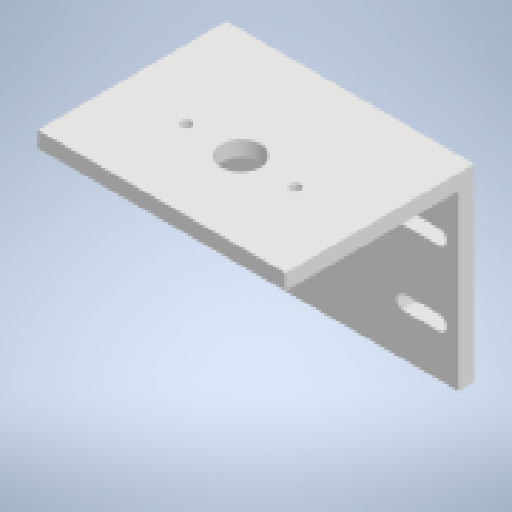
# Autodesk Inventor part: Suporte motor sensor
Saved by Autodesk Inventor 2023 (Build 270158000, 158)
## iProperties
Created: 2022-10-13
Part Number: Suporte motor sensor
Material: Generic
Document SubType Name: Modeling
Designer: klebe
Density: 1 g/cm^3
Appearance: Default
Author: klebe
Autodesk Inventor part; units mm, degrees
ref_plane "YZ Plane" through (0, 0, 0) normal (1, 0, 0) x (0, 1, 0)
ref_plane "XZ Plane" through (0, 0, 0) normal (0, 1, 0) x (-1, 0, 0)
ref_plane "XY Plane" through (0, 0, 0) normal (0, 0, 1) x (1, 0, 0)
sketch "Sketch1" plane through (0, 0, 0) normal (0, 0, 1) x (1, 0, 0)
  line L0 (-200, 100) -> (200, 100) projected
  line L1 (-200, -100) -> (-200, 100) projected
  line L2 (200, -100) -> (-200, -100) projected
  line L3 (121.9, 74) -> (121.9, 71)
  line L4 (171.9, 74) -> (121.9, 74)
  line L5 (171.9, 71) -> (171.9, 35.9)
  line L6 (121.9, 71) -> (171.9, 71)
  line L7 (121.9, 71) -> (121.9, 35.9)
  line L8 (171.9, 35.9) -> (121.9, 35.9)
  line L9 (171.9, 71) -> (171.9, 35.9)
  line L10 (171.9, 74) -> (171.9, 71)
  line L11 (121.9, 35.9) -> (171.9, 35.9)
  line L12 (171.9, 35.9) -> (171.9, 71)
  line L13 (171.9, 71) -> (121.9, 71)
  line L14 (121.9, 71) -> (121.9, 35.9)
  point P0 (0, 0)
  constraints: 24 end point, 2 parallel, 1 horizontal, 1 perpendicular
extrude "Extrusion1" add sketch "Sketch1" along normal blind 3.175
sketch "Sketch2" plane through (0, 0, 3.175) normal (0, 0, 1) x (1, 0, 0)
  line L0 (171.9, 74) -> (121.9, 74) projected
  line L1 (171.9, 35.9) -> (171.9, 74) projected
  line L2 (121.9, 74) -> (171.9, 74)
  line L3 (171.9, 74) -> (171.9, 71)
  line L4 (121.9, 71) -> (121.9, 74)
  line L5 (121.9, 71) -> (121.9, 70.825)
  line L6 (121.9, 74) -> (121.9, 35.9) projected
  line L7 (121.9, 70.825) -> (171.9, 70.825)
  line L8 (171.9, 71) -> (171.9, 70.825)
  line L9 (171.9, 71) -> (171.9, 70.825)
  point P0 (0, 0)
  dimension "d3" = 3
  dimension "d54" = 0.175
  constraints: 14 end point, 3 point on line, 2 collinear, 2 perpendicular, 1 horizontal, 1 parallel
  measures "d3" distance of L2.end L3.end
  measures "d54" distance of L4.start L5.end
extrude "Extrusion2" add sketch "Sketch2" along normal blind 34.925
sketch "Sketch3" plane through (121.9, 74, 0) normal (0, 1, 0) x (1, 0, 0)
  line L0 (50, 0) -> (0, 0) projected
  line L1 (0, 0) -> (0, -38.1) projected
  line L2 (50, -38.1) -> (0, -38.1) projected
  line L3 (50, 0) -> (50, -38.1) projected
  line L4 (50, -3.175) -> (50, -38.1) projected
  line L5 (0, -38.1) -> (0, -19.225)
  line L6 (50, -19.05) -> (60.9839, -19.05)
  line L7 (0, -38.1) -> (0, -22.1)
  line L8 (0, -22.1) -> (14, -22.1)
  line L9 (36, -22.1) -> (36, -22)
  point P0 (-121.9, 0)
  point P1 (14, -22)
  dimension "d55" = 16
  constraints: 10 end point, 4 point on line, 2 perpendicular, 1 vertical
  measures "d55" distance of L1.end L7.end
sketch "Sketch4" plane through (121.9, 74, 0) normal (0, 1, 0) x (1, 0, 0)
  line L0 (50, 0) -> (0, 0) projected
  line L1 (0, 0) -> (0, -38.1) projected
  line L2 (50, -38.1) -> (0, -38.1) projected
  line L3 (50, 0) -> (50, -38.1) projected
  line L4 (0, -38.1) -> (0, -22.1)
  line L5 (25, -22) -> (25, -22)
  point P0 (-121.9, 0)
  dimension "d56" = 16
  constraints: 4 end point, 1 point on line, 1 vertical
  measures "d56" distance of L1.end L4.end
hole "Hole2" at (146.9, 74, 22) direction (0, -1, 0) diameter 8 end through all
hole "Hole3" at (135.9, 74, 22.1) at (157.9, 74, 22.1) direction (0, -1, 0) diameter 2 end through all
sketch "Sketch5" plane through (0, 0, 3.175) normal (0, 0, 1) x (1, 0, 0)
  line L0 (121.9, 70.825) -> (121.9, 35.9) projected
  line L1 (121.9, 35.9) -> (171.9, 35.9) projected
  line L2 (171.9, 35.9) -> (171.9, 70.825) projected
  line L3 (171.9, 70.825) -> (121.9, 70.825) projected
  line L4 (121.9, 35.9) -> (171.9, 35.9) projected
  line L5 (171.9, 35.9) -> (167.9, 35.9)
  arc A0 (167.9, 44.31) -> (167.9, 47.49) centre (167.9, 45.9) ccw
  arc A1 (160.9, 47.49) -> (160.9, 44.31) centre (160.9, 45.9) ccw
  line L6 (167.9, 44.31) -> (160.9, 44.31)
  line L7 (160.9, 47.49) -> (167.9, 47.49)
  arc A2 (167.9, 59.31) -> (167.9, 62.49) centre (167.9, 60.9) ccw
  arc A3 (160.9, 62.49) -> (160.9, 59.31) centre (160.9, 60.9) ccw
  line L8 (167.9, 59.31) -> (160.9, 59.31)
  line L9 (160.9, 62.49) -> (167.9, 62.49)
  arc A4 (132.9, 44.31) -> (132.9, 47.49) centre (132.9, 45.9) ccw
  arc A5 (125.9, 47.49) -> (125.9, 44.31) centre (125.9, 45.9) ccw
  line L10 (132.9, 44.31) -> (125.9, 44.31)
  line L11 (125.9, 47.49) -> (132.9, 47.49)
  arc A6 (132.9, 59.31) -> (132.9, 62.49) centre (132.9, 60.9) ccw
  arc A7 (125.9, 62.49) -> (125.9, 59.31) centre (125.9, 60.9) ccw
  line L12 (132.9, 59.31) -> (125.9, 59.31)
  line L13 (125.9, 62.49) -> (132.9, 62.49)
  point P0 (0, 0)
  constraints: 18 end point, 16 point on circle, 12 tangent, 8 centre point, 1 point on line
extrude "Extrusion3" cut sketch "Sketch5" against normal blind 4 contours L6 A1 L7 A0 | L8 A3 L9 A2 | L10 A5 L11 A4 | L12 A7 L13 A6
body "Solid1"
